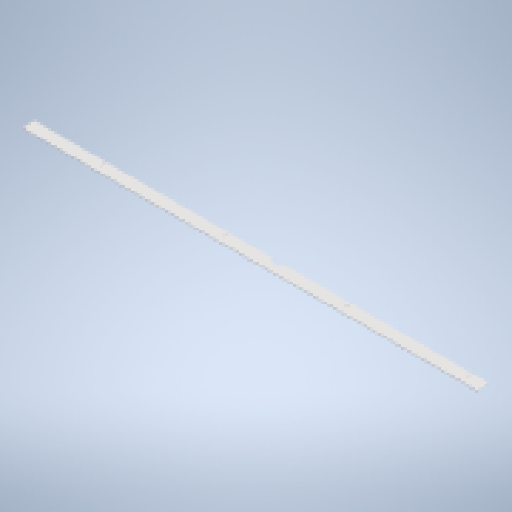
# Autodesk Inventor part: BSH 033 stringer floor 3
Saved by Autodesk Inventor 2025 (Build 290162010, 162A)
## iProperties
Created: 2024-07-23
Part Number: BSH 033 stringer floor 3
Material: 09g2s
Document SubType Name: Sheet Metal
Designer: admin
Stock Number: БШК 032 стрингер пол 2
Mass: 5330.4 g
Surface Area: 4696.25 cm^2
Volume: 679.031 cm^3
Density: 7.85 g/cm^3
Flat Pattern Width: 5 cm
Flat Pattern Length: 186 cm
Flat Pattern Area: 930 cm^2
Sheet Metal Rule: AISI304 3mm Die 32
Sheet Metal Width: 50,000 mm
Sheet Metal Length: 1860,000 mm
Sheet Metal Area: 93000,000 mm^2
Appearance: Default
Author: admin
Autodesk Inventor part; units mm, degrees
ref_plane "YZ Plane" through (0, 0, 0) normal (1, 0, 0) x (0, 1, 0)
ref_plane "XZ Plane" through (0, 0, 0) normal (0, 1, 0) x (-1, 0, 0)
ref_plane "XY Plane" through (0, 0, 0) normal (0, 0, 1) x (1, 0, 0)
sketch "Sketch8" plane through (0, 0, 0) normal (0, 0, 1) x (1, 0, 0)
  line L0 (-930, 50) -> (930, 50)
  line L1 (930, 50) -> (930, 0)
  line L2 (930, 0) -> (-930, 0)
  line L3 (-930, 0) -> (-930, 50)
  point P0 (0, 0)
  point P1 (0, 0)
  dimension "d37" = 50
  dimension "d38" = 1860
  measures "d37" distance of L0.end L1.end
  measures "d38" distance of L0.start L0.end
extrude "Plate5" add sketch "Sketch8" against normal blind 3
sketch "Sketch9" plane through (0, 0, 0) normal (0, 0, 1) x (1, 0, 0)
  line L0 (930, 50) -> (-930, 50) projected
  line L1 (-784, 50) -> (-780.8, 50)
  line L2 (-780.8, 50) -> (-780.8, 24)
  line L3 (-780.8, 24) -> (-784, 24)
  line L4 (-784, 24) -> (-784, 50)
  line L5 (-930, 50) -> (-930, 0) projected
  point P0 (0, 0)
  point P1 (-780.8, 50)
  dimension "d42" = 146
  dimension "d43" = 3.2
  dimension "d44" = 26
  constraints: 8 end point, 2 parallel, 1 horizontal, 1 perpendicular, 1 point on line
  measures "d42" distance between parallel lines of L4 L5
  measures "d43" distance between parallel lines of L4 L2
  measures "d44" distance of L1.end L2.end
extrude "Extrusion3" cut sketch "Sketch9" against normal through all
pattern_linear "Rectangular Pattern2" count 6 spacing 500 along (1, 0, 0) of "Extrusion3"
sketch "Sketch10" plane through (0, 0, 0) normal (0, 0, 1) x (1, 0, 0)
  line L0 (930, 50) -> (719.2, 50) projected
  line L1 (719.2, 50) -> (719.2, 24) projected
  line L2 (719.2, 24) -> (716, 24) projected
  line L3 (716, 24) -> (716, 50) projected
  line L4 (716, 50) -> (219.2, 50) projected
  line L5 (219.2, 50) -> (219.2, 24) projected
  line L6 (219.2, 24) -> (216, 24) projected
  line L7 (216, 24) -> (216, 50) projected
  line L8 (216, 50) -> (-280.8, 50) projected
  line L9 (-280.8, 50) -> (-280.8, 24) projected
  line L10 (-280.8, 24) -> (-284, 24) projected
  line L11 (-284, 24) -> (-284, 50) projected
  line L12 (-284, 50) -> (-780.8, 50) projected
  line L13 (-780.8, 50) -> (-780.8, 24) projected
  line L14 (-780.8, 24) -> (-784, 24) projected
  line L15 (-784, 24) -> (-784, 50) projected
  line L16 (-784, 50) -> (-930, 50) projected
  line L17 (-930, 50) -> (-930, 0) projected
  line L18 (-930, 0) -> (930, 0) projected
  line L19 (930, 0) -> (930, 50) projected
  circle A0 centre (440, 50) radius 20
  point P0 (0, 0)
  point P1 (420, 50)
  point P2 (460, 50)
  point P3 (50, 50)
  point P4 (90, 50)
  dimension "d50" = 40
  dimension "d52" = 1370
  constraints: 2 point on line, 1 centre point
  measures "d50" diameter of A0
  measures "d52" distance from line of L17 A0.centre
extrude "Extrusion4" cut sketch "Sketch10" against normal through all contours A0 L4 | L4 A0
sketch "Sketch11" plane through (0, 0, 0) normal (0, 0, 1) x (1, 0, 0)
  line L0 (-752.5883, 29.3223) -> (-521.0772, 29.3223) construction
  line L1 (-521.0772, 29.3223) -> (-521.0772, 13.038) construction
  line L2 (-521.0772, 13.038) -> (-752.5883, 13.038) construction
  line L3 (-752.5883, 13.038) -> (-752.5883, 29.3223) construction
  point P0 (0, 0)
  constraints: 2 other
mark "Mark1"
equation "\"d41\" = Thickness"
equation "\"BendReliefWidth\" = Thickness"
equation "\"BendReliefDepth\" = 0.5 * Thickness"
equation "\"CornerReliefSize\" = 4 * Thickness"
equation "\"MinimumRemnant\" = 2 * Thickness"
equation "\"TransitionRadius\" = BendRadius"
equation "\"JacobiRadiusSize\" = BendRadius"
equation "\"GapSize\" = Thickness"
equation "\"Thickness\" = 3"
equation "\"BendRadius\" = 5"
body "Solid3"
